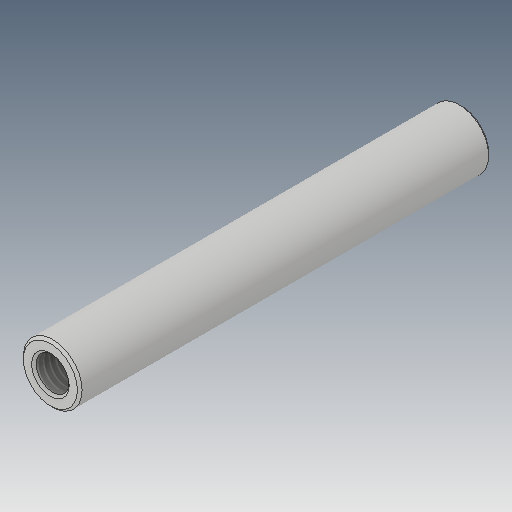
# Autodesk Inventor part: Frame Spacer
Saved by Autodesk Inventor 2018 (Build 220112000, 112)
## iProperties
Created: 2018-01-03
Part Number: Frame Spacer
Material: Generic
Document SubType Name: Modeling
Designer: fbl92568
Density: 1 g/cm^3
Appearance: Default
Mass: 0.47073 g
Surface Area: 8.78868 cm^2
Volume: 0.47073 cm^3
Author: fbl92568
Autodesk Inventor part; units mm, degrees
ref_plane "YZ Plane" through (0, 0, 0) normal (1, 0, 0) x (0, 1, 0)
ref_plane "XZ Plane" through (0, 0, 0) normal (0, 1, 0) x (-1, 0, 0)
ref_plane "XY Plane" through (0, 0, 0) normal (0, 0, 1) x (1, 0, 0)
sketch "Sketch1" plane through (0, 0, 0) normal (0, 0, 1) x (1, 0, 0)
  circle A0 centre (0, 0) radius 2.5
  circle A1 centre (0, 0) radius 1.4
  dimension "d0" = 5
  dimension "d1" = 2.8
  constraints: 2 centre point, 2 coincident
  measures "d0" diameter of A0
  measures "d1" diameter of A1
extrude "Extrusion1" add sketch "Sketch1" along normal blind 35
thread "Thread1" size "M3x0.5" class "6H" standard "ANSI Metric M Profile" length 10
thread "Thread2" size "M3x0.5" class "6H" standard "ANSI Metric M Profile" length 10
chamfer "Chamfer1" distance 0.2 angle 45 4 edges at (-1.4, 0, 0) (-2.5, 0, 0) (-1.4, 0, 35) (-2.5, 0, 35)
body "Solid1"
